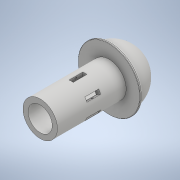
# Autodesk Inventor part: 主體
Saved by Autodesk Inventor 2020 (Build 240168000, 168)
## iProperties
Created: 2021-03-05
Part Number: 主體
Material: 一般
Document SubType Name: Modeling
Designer: 王鼎鈞
Density: 1 g/cm^3
Appearance: 預設
Mass: 319.933 g
Surface Area: 399.291 cm^2
Volume: 319.933 cm^3
Author: 王鼎鈞
Autodesk Inventor part; units mm, degrees
ref_plane "YZ Plane" through (0, 0, 0) normal (1, 0, 0) x (0, 1, 0)
ref_plane "XZ Plane" through (0, 0, 0) normal (0, 1, 0) x (-1, 0, 0)
sketch "草圖1" plane through (0, 0, 0) normal (1, 0, 0) x (0, 1, 0)
  line L0 (0, 0) -> (100, 0)
  line L1 (100, 0) -> (100, -25)
  line L2 (100, -25) -> (0, -25)
  line L3 (0, -25) -> (0, 0)
  dimension "d0" = 100
  dimension "d1" = 25
  constraints: 8 end point, 2 parallel, 1 horizontal, 1 perpendicular
  measures "d0" distance of L1.end L2.end
  measures "d1" distance of L0.end L1.end
revolve "迴轉1" add sketch "草圖1" angle 360 about axis through (0, 0, 0) along (0, 1, 0)
sketch "草圖2" plane through (0, 0, 0) normal (1, 0, 0) x (0, 1, 0)
  line L0 (100, 25) -> (100, -25) projected
  line L1 (100, 0) -> (105, 0)
  line L2 (105, 0) -> (105, 45)
  line L3 (105, 45) -> (100, 45)
  line L4 (100, 45) -> (100, 0)
  point P0 (0, 0)
  dimension "d3" = 5
  dimension "d4" = 45
  constraints: 8 end point, 2 parallel, 1 horizontal, 1 midpoint, 1 perpendicular
  measures "d3" distance of L3.end L2.end
  measures "d4" distance of L2.end L1.end
revolve "迴轉2" add sketch "草圖2" angle 360 about axis through (0, 100, 0) along (0, 1, 0)
fillet "圓角1" radius 3 1 edges at (0, 105, -45)
fillet "圓角2" radius 0.5 1 edges at (0, 100, -45)
sketch "草圖3" plane through (0, 0, 0) normal (1, 0, 0) x (0, 1, 0)
  line L0 (105, 42) -> (105, -42)
  arc A0 (144.882585, 0) -> (105, 39.882585) centre (105, 0) ccw
  line L1 (144.882585, 0) -> (105, 0)
  point P0 (0, 0)
  constraints: 2 end point, 2 point on circle, 1 centre point, 1 midpoint, 1 perpendicular, 1 point on line
revolve "迴轉3" add sketch "草圖3" angle 360 about axis through (0, 144.882585, 0) along (0, -1, 0)
sketch "草圖4" plane through (0, 0, 0) normal (0, -1, 0) x (1, 0, 0)
  circle A0 centre (0, 0) radius 17.5
  dimension "d9" = 35
  constraints: 1 centre point, 1 coincident
  measures "d9" diameter of A0
extrude "擠出1" cut sketch "草圖4" against normal blind 40
sketch "草圖5" plane through (0, 0, 0) normal (1, 0, 0) x (0, 1, 0)
  line L0 (0, 25) -> (0, -25)
  line L1 (100, 25) -> (100, -25)
  line L2 (100, 25) -> (0, 25)
  arc A0 (53.348624, 19.495413) -> (56.651376, 19.495413) centre (55, 22) ccw
  line L3 (65, 25) -> (56.651376, 19.495413)
  line L4 (45, 25) -> (53.348624, 19.495413)
  circle A1 centre (55, 22) radius 1.5
  line L5 (65, 25) -> (65, 35.07297)
  line L6 (65, 35.07297) -> (43.500596, 35.585049)
  line L7 (43.500596, 35.585049) -> (45, 25)
  point P0 (0, 0)
  dimension "d12" = 6
  dimension "d13" = 0
  dimension "d14" = 55
  dimension "d15" = 10
  dimension "d16" = 10
  dimension "d17" = 3
  constraints: 10 end point, 2 centre point, 2 point on circle, 2 point on line, 2 tangent, 1 coincident, 1 vertical
  measures "d12" diameter of A0
  measures "d13" distance edge to line of A0 L2
  measures "d14" distance from line of L0 A0.centre
  measures "d15" horizontal distance of A0.centre L4.start
  measures "d16" horizontal distance of A0.centre L3.start
  measures "d17" diameter of A1
extrude "擠出2" cut sketch "草圖5" along normal mid plane 6
pattern_circular "環形陣列1" count 6 over 360 about axis through (0, -10, 0) along (0, 1, 0) of "擠出2"
sketch "草圖7" plane through (0, 0, 0) normal (1, 0, 0) x (0, 1, 0)
  line L0 (-28.970873, 0) -> (173.82524, 0)
  line L1 (0, -63) -> (0, 63)
  line L2 (40, -17.5) -> (40, 17.5)
  line L3 (107.858315, 0) -> (40, 0)
  line L4 (40, 0) -> (40, 17.5)
  line L5 (40, 17.5) -> (107.858315, 17.5)
  line L6 (107.858315, 17.5) -> (107.858315, 0)
  point P0 (0, 0)
  constraints: 8 end point, 2 parallel, 1 horizontal, 1 perpendicular, 1 point on line
revolve "迴轉4" cut sketch "草圖7" angle 360 about axis through (0, -10, 0) along (0, 1, 0)
sketch "草圖8" plane through (0, 0, 0) normal (1, 0, 0) x (0, 1, 0)
  ellipse E0 centre (82.916667, 0) end of major axis (119.884476, -17.000422) minor radius 20.17524 (45.27399, 15.00775) -> (45.27399, 9.811597) ccw
  line L0 (45.27399, 9.811597) -> (64.72601, 9.811597)
  ellipse E1 centre (27.083333, 0) end of major axis (-9.884476, -17.000422) minor radius 20.17524 (64.72601, 9.811597) -> (64.72601, 15.00775) ccw
  line L1 (64.72601, 15.00775) -> (45.27399, 15.00775)
  ellipse E2 centre (82.916667, 0) end of major axis (45.948857, -17.000422) minor radius 20.17524 (45.27399, -9.811597) -> (45.27399, -15.00775) ccw
  line L2 (45.27399, -15.00775) -> (64.72601, -15.00775)
  ellipse E3 centre (27.083333, 0) end of major axis (64.051143, -17.000422) minor radius 20.17524 (64.72601, -15.00775) -> (64.72601, -9.811597) ccw
  line L3 (64.72601, -9.811597) -> (45.27399, -9.811597)
  line L4 (45.27399, -24.819347) -> (45.27399, -24.819347)
  line L5 (45.27399, -24.819347) -> (64.72601, -24.819347)
  line L6 (64.72601, -24.819347) -> (64.72601, -24.819347)
  line L7 (64.72601, -24.819347) -> (45.27399, -24.819347)
  ellipse E4 centre (82.916667, 0) end of major axis (45.948857, -17.000422) minor radius 20.17524 (45.27399, -9.811597) -> (45.27399, -15.00775) ccw
  line L8 (45.27399, -9.811597) -> (64.72601, -9.811597)
  ellipse E5 centre (27.083333, 0) end of major axis (64.051143, -17.000422) minor radius 20.17524 (64.72601, -15.00775) -> (64.72601, -9.811597) ccw
  line L9 (64.72601, -15.00775) -> (45.27399, -15.00775)
  ellipse E6 centre (82.916667, 0) end of major axis (119.884476, -17.000422) minor radius 20.17524 (45.27399, 15.00775) -> (45.27399, 9.811597) ccw
  line L10 (45.27399, 15.00775) -> (64.72601, 15.00775)
  ellipse E7 centre (27.083333, 0) end of major axis (-9.884476, -17.000422) minor radius 20.17524 (64.72601, 9.811597) -> (64.72601, 15.00775) ccw
  line L11 (64.72601, 9.811597) -> (45.27399, 9.811597)
  line L12 (45.27399, 24.819347) -> (45.27399, 24.819347)
  line L13 (45.27399, 24.819347) -> (64.72601, 24.819347)
  line L14 (64.72601, 24.819347) -> (64.72601, 24.819347)
  line L15 (64.72601, 24.819347) -> (45.27399, 24.819347)
  line L16 (0, 25) -> (0, -25)
  line L17 (100, 25) -> (100, -25)
  line L18 (100, -25) -> (0, -25)
  ellipse E8 centre (27.083333, 0) end of major axis (64.051143, -17.000422) minor radius 20.17524 (64.72601, -15.00775) -> (64.72601, -9.811597) ccw
  line L19 (45.001312, -25) -> (64.995309, -25)
  line L20 (64.995309, -25) -> (64.995309, -12.157897)
  line L21 (64.995309, -12.157897) -> (45.001312, -12.157897)
  line L22 (45.001312, -12.157897) -> (45.001312, -25)
  circle A0 centre (55, -22) radius 1.5
  circle A1 centre (55, -22) radius 1.5
  point P0 (0, 0)
  constraints: 8 end point, 2 parallel, 1 horizontal, 1 perpendicular, 1 point on line, 10 other
sketch "草圖8 outline for 擠出4" plane through (0, 0, 0) normal (1, 0, 0) x (0, 1, 0)
  line L0 (64.995309, -25) -> (64.995309, -12.157897)
  line L1 (45.001312, -25) -> (64.995309, -25)
  line L2 (64.995309, -12.157897) -> (45.001312, -12.157897)
  line L3 (45.001312, -12.157897) -> (45.001312, -25)
  circle A0 centre (55, -22) radius 1.5
extrude "擠出4" cut sketch "草圖8 outline for 擠出4" along normal mid plane 6
pattern_circular "環形陣列2" count 6 over 360 about axis through (0, -10, 0) along (0, 1, 0) of "擠出4"
sketch "草圖9" plane through (0, 0, 0) normal (1, 0, 0) x (0, 1, 0)
  circle A0 centre (55, -22) radius 1.5
  circle A1 centre (55, -22) radius 18.5
  circle A2 centre (55, 22) radius 1.5
  circle A3 centre (55, 22) radius 18.5
  line L0 (0, -17.5) -> (107.858315, -17.5)
  line L1 (0, 17.5) -> (107.858315, 17.5)
  line L2 (81.619047, -17.5) -> (31.619047, -17.5)
  line L3 (31.619047, -17.5) -> (31.619047, 17.5)
  line L4 (31.619047, 17.5) -> (81.619047, 17.5)
  line L5 (81.619047, 17.5) -> (81.619047, -17.5)
  point P0 (0, 0)
  dimension "d33" = 37
  dimension "d34" = 37
  dimension "d35" = 50
  constraints: 8 end point, 2 centre point, 2 coincident, 2 parallel, 2 point on line, 1 horizontal, 1 perpendicular
  measures "d33" diameter of A1
  measures "d34" diameter of A3
  measures "d35" distance between parallel lines of L5 L3
ref_plane "工作平面1" through (0, 0, 0) normal (1, 0, 0) x (0, 0, -1)
sketch "草圖10" plane through (0, 0, 0) normal (1, 0, 0) x (0, 0, -1)
  line L0 (24.819347, 64.995309) -> (24.819347, 45.001312)
  line L1 (24.819347, 45.001312) -> (24.999135, 45.001312)
  line L2 (24.999135, 45.001312) -> (24.999135, 45.001312)
  line L3 (24.999135, 45.001312) -> (24.819347, 45.001312)
  line L4 (24.819347, 45.001312) -> (24.819347, 64.995309)
  line L5 (24.819347, 64.995309) -> (24.996907, 64.995309)
  line L6 (24.996907, 64.995309) -> (24.996907, 64.995309)
  line L7 (24.996907, 64.995309) -> (24.819347, 64.995309)
  line L8 (-25, 0) -> (25, 0)
  line L9 (-25, 100) -> (25, 100)
  line L10 (12.157897, 64.995309) -> (9.811597, 64.995309)
  line L11 (9.811597, 64.995309) -> (9.811597, 45.001312)
  line L12 (9.811597, 45.001312) -> (12.319447, 45.001312)
  ellipse E0 centre (0, 82.916667) end of major axis (17.000422, 45.948857) minor radius 20.17524 (12.319447, 45.001312) -> (12.679688, 45.001312) ccw
  line L13 (12.679688, 45.001312) -> (15.00775, 45.001312)
  line L14 (15.00775, 45.001312) -> (15.00775, 64.995309)
  line L15 (15.00775, 64.995309) -> (12.83901, 64.995309)
  ellipse E1 centre (0, 27.083333) end of major axis (17.000422, 64.051143) minor radius 20.17524 (12.83901, 64.995309) -> (12.157897, 64.995309) ccw
  line L16 (-12.83901, 64.995309) -> (-15.00775, 64.995309)
  line L17 (-15.00775, 64.995309) -> (-15.00775, 45.001312)
  line L18 (-15.00775, 45.001312) -> (-12.679688, 45.001312)
  ellipse E2 centre (0, 82.916667) end of major axis (17.000422, 119.884476) minor radius 20.17524 (-12.679688, 45.001312) -> (-12.319447, 45.001312) ccw
  line L19 (-12.319447, 45.001312) -> (-9.811597, 45.001312)
  line L20 (-9.811597, 45.001312) -> (-9.811597, 64.995309)
  line L21 (-9.811597, 64.995309) -> (-12.157897, 64.995309)
  ellipse E3 centre (0, 27.083333) end of major axis (17.000422, -9.884476) minor radius 20.17524 (-12.157897, 64.995309) -> (-12.83901, 64.995309) ccw
  line L22 (-24.996907, 64.995309) -> (-24.819347, 64.995309)
  line L23 (-24.819347, 64.995309) -> (-24.819347, 45.001312)
  line L24 (-24.819347, 45.001312) -> (-24.999135, 45.001312)
  line L25 (-24.999135, 45.001312) -> (-24.999135, 45.001312)
  line L26 (-24.999135, 45.001312) -> (-24.819347, 45.001312)
  line L27 (-24.819347, 45.001312) -> (-24.819347, 64.995309)
  line L28 (-24.819347, 64.995309) -> (-24.996907, 64.995309)
  line L29 (-24.996907, 64.995309) -> (-24.996907, 64.995309)
  line L30 (-12.157897, 64.995309) -> (-9.811597, 64.995309)
  line L31 (-9.811597, 64.995309) -> (-9.811597, 45.001312)
  line L32 (-9.811597, 45.001312) -> (-12.319447, 45.001312)
  ellipse E4 centre (0, 82.916667) end of major axis (17.000422, 119.884476) minor radius 20.17524 (-12.679688, 45.001312) -> (-12.319447, 45.001312) ccw
  line L33 (-12.679688, 45.001312) -> (-15.00775, 45.001312)
  line L34 (-15.00775, 45.001312) -> (-15.00775, 64.995309)
  line L35 (-15.00775, 64.995309) -> (-12.83901, 64.995309)
  ellipse E5 centre (0, 27.083333) end of major axis (17.000422, -9.884476) minor radius 20.17524 (-12.157897, 64.995309) -> (-12.83901, 64.995309) ccw
  line L36 (12.83901, 64.995309) -> (15.00775, 64.995309)
  line L37 (15.00775, 64.995309) -> (15.00775, 45.001312)
  line L38 (15.00775, 45.001312) -> (12.679688, 45.001312)
  ellipse E6 centre (0, 82.916667) end of major axis (17.000422, 45.948857) minor radius 20.17524 (12.319447, 45.001312) -> (12.679688, 45.001312) ccw
  line L39 (12.319447, 45.001312) -> (9.811597, 45.001312)
  line L40 (9.811597, 45.001312) -> (9.811597, 64.995309)
  line L41 (9.811597, 64.995309) -> (12.157897, 64.995309)
  ellipse E7 centre (0, 27.083333) end of major axis (17.000422, 64.051143) minor radius 20.17524 (12.83901, 64.995309) -> (12.157897, 64.995309) ccw
  circle A0 centre (-22, 55) radius 1.5
  point P0 (0, 0)
  constraints: 8 other
extrude "擠出5" cut sketch "草圖10" along normal mid plane 8 contours A0
pattern_circular "環形陣列3" count 6 over 360 about axis through (0, 50, 0) along (0, -1, 0) of "擠出5"
